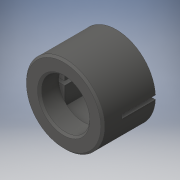
# Autodesk Inventor part: MagnetHolder
Saved by Autodesk Inventor 2016 (Build 200138000, 138)
## iProperties
Created: 2016-11-06
Part Number: MagnetHolder
Material: Generic
Document SubType Name: Modeling
Designer: brent
Density: 1 g/cm^3
Appearance: Default
Author: brent
Autodesk Inventor part; units mm, degrees
ref_plane "YZ Plane" through (0, 0, 0) normal (1, 0, 0) x (0, 1, 0)
ref_plane "XZ Plane" through (0, 0, 0) normal (0, 1, 0) x (-1, 0, 0)
ref_plane "XY Plane" through (0, 0, 0) normal (0, 0, 1) x (1, 0, 0)
sketch "Sketch1" plane through (0, 0, 0) normal (0, 0, 1) x (1, 0, 0)
  line L0 (-2.375, 2.5709) -> (-2.375, -2.5709) projected
  arc A0 (-2.375, -2.5709) -> (2.375, -2.5709) centre (0, 0) ccw projected
  line L1 (2.375, -2.5709) -> (2.375, 2.5709) projected
  arc A1 (2.375, 2.5709) -> (-2.375, 2.5709) centre (0, 0) ccw projected
  circle A2 centre (0, 0) radius 0.875 projected
  circle A3 centre (0, 0) radius 5
  dimension "d0" = 10
  constraints: 1 centre point, 1 coincident
  measures "d0" diameter of A3
ref_plane "Work Plane1" through (-2.375, -3.5, 4.25) normal (0, 0, 1) x (1, 0, 0)
extrude "Extrusion1" add sketch "Sketch1" along normal up to surface (4.25 mm away) contours A3
sketch "Sketch2" plane through (0, 0, 4.25) normal (0, 0, 1) x (1, 0, 0)
  circle A0 centre (0, 0) radius 3.1
  circle A1 centre (0, 0) radius 5 projected
  dimension "d3" = 6.2
  constraints: 1 centre point, 1 coincident
  measures "d3" diameter of A0
extrude "Extrusion2" add sketch "Sketch2" along normal blind 2.5
sketch "Sketch3" plane through (0, 0, 0) normal (0, 0, -1) x (-1, 0, 0)
  line L0 (-5.064, 0) -> (5.064, 0) construction
  line L1 (-5.064, -0.25) -> (5.064, -0.25)
  line L2 (5.064, 0.25) -> (-5.064, 0.25)
  arc A0 (-5.064, 0.25) -> (-5.064, -0.25) centre (-5.064, 0) ccw
  arc A1 (5.064, -0.25) -> (5.064, 0.25) centre (5.064, 0) ccw
  point P0 (0, 0)
  dimension "d6" = 0.5
  constraints: 8 end point, 4 point on circle, 4 tangent, 2 centre point, 1 horizontal, 1 midpoint, 1 parallel
  measures "d6" diameter of A1
extrude "Extrusion3" cut sketch "Sketch3" against normal blind 4.25
chamfer "Chamfer1" distance 0.25 angle 45 2 edges at (-3.1, 0, 6.75) (-5, 0, 6.75)
body "Solid1"
